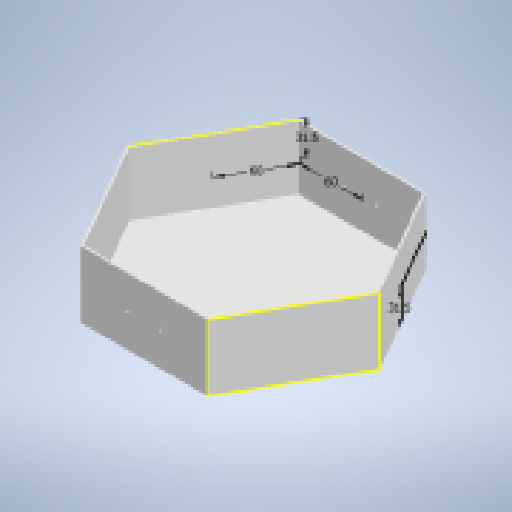
# Autodesk Inventor part: BaseHEX
Saved by Autodesk Inventor 2024 (Build 280153000, 153)
## iProperties
Created: 2024-03-21
Part Number: BaseHEX
Material: Genérico
Document SubType Name: Modeling
Designer: na_re
Density: 1 g/cm^3
Appearance: Valor por defecto
Author: na_re
Autodesk Inventor part; units mm, degrees
ref_plane "YZ Plane" through (0, 0, 0) normal (1, 0, 0) x (0, 1, 0)
ref_plane "XZ Plane" through (0, 0, 0) normal (0, 1, 0) x (-1, 0, 0)
ref_plane "XY Plane" through (0, 0, 0) normal (0, 0, 1) x (1, 0, 0)
sketch "Boceto1" plane through (0, 0, 0) normal (0, 1, 0) x (-1, 0, 0)
  line L0 (120, 0) -> (60, -103.923)
  line L1 (60, -103.923) -> (-60, -103.923)
  line L2 (-60, -103.923) -> (-120, 0)
  line L3 (-120, 0) -> (-60, 103.923)
  line L4 (-60, 103.923) -> (60, 103.923)
  line L5 (60, 103.923) -> (120, 0)
  point P0 (0, 0)
  point P1 (0, 0)
  dimension "d0" = 120
  constraints: 12 end point, 1 coincident, 13 other
  measures "d0" distance of L0.start L0.end
extrude "Extrusión1" add sketch "Boceto1" along normal blind 3
sketch "Boceto2" plane through (0, 3, 0) normal (0, 1, 0) x (1, 0, 0)
  line L0 (-60, -103.923) -> (60, -103.923) projected
  line L1 (60, -103.923) -> (120, 0) projected
  line L2 (120, 0) -> (60, 103.923) projected
  line L3 (60, 103.923) -> (-60, 103.923) projected
  line L4 (-60, 103.923) -> (-120, 0) projected
  line L5 (-120, 0) -> (-60, -103.923) projected
  line L6 (-58.8453, -101.923) -> (58.8453, -101.923)
  line L7 (58.8453, -101.923) -> (117.6906, 0)
  line L8 (117.6906, 0) -> (58.8453, 101.923)
  line L9 (58.8453, 101.923) -> (-58.8453, 101.923)
  line L10 (-58.8453, 101.923) -> (-117.6906, 0)
  line L11 (-117.6906, 0) -> (-58.8453, -101.923)
  point P0 (0, 0)
  dimension "d3" = 2
  constraints: 12 end point, 5 other
  measures "d3" distance between parallel lines of L5 L11
extrude "Extrusión2" add sketch "Boceto2" along normal blind 60
sketch "Boceto5" plane through (120, 0, 0) normal (0.866, 0, 0.5) x (0.5, 0, -0.866)
  line L0 (-120, 0) -> (0, 0) projected
  line L1 (0, 0) -> (0, 63) projected
  line L2 (-120, 63) -> (0, 63) projected
  line L3 (-120, 0) -> (-120, 63) projected
  point P0 (-60, 0)
sketch "Boceto9" plane through (-60, 0, 103.923) normal (-0.866, 0, 0.5) x (0.5, 0, 0.866)
  circle A0 centre (-117, 58.5) radius 1.5 projected
  circle A1 centre (-3, 58.5) radius 1.5 projected
  point P0 (-60, 0)
extrude "Extrusión7" cut sketch "Boceto9" against normal blind 220
sketch "Boceto10" plane through (-120, 0, 0) normal (-0.866, 0, -0.5) x (-0.5, 0, 0.866)
  line L0 (-120, 0) -> (0, 0) projected
  line L1 (0, 0) -> (0, 63) projected
  line L2 (-120, 63) -> (0, 63) projected
  line L3 (-120, 0) -> (-120, 63) projected
  line L4 (-120, 63) -> (-120, 31.5)
  line L5 (-120, 31.5) -> (-60, 31.5)
  line L6 (-60, 31.5) -> (-60, 0)
  dimension "d19" = 31.5
  dimension "d20" = 60
  constraints: 6 end point, 1 midpoint, 1 perpendicular
  measures "d19" distance of L2.start L4.end
  measures "d20" distance of L4.end L5.end
sketch "Boceto12" plane through (60, 0, -103.923) normal (0, 0, -1) x (-1, 0, 0)
  line L0 (120, 0) -> (120, 63) projected
  line L1 (120, 31.5) -> (60, 31.5)
  line L2 (60, 31.5) -> (60, 0)
  dimension "d23" = 60
  constraints: 4 end point, 1 horizontal, 1 midpoint
  measures "d23" distance of L1.start L1.end
sketch "Boceto13" plane through (60, 0, -103.923) normal (0, 0, -1) x (-1, 0, 0)
  circle A0 centre (44.5, 31.5) radius 1.25 projected
  circle A1 centre (75.5, 31.5) radius 1.25 projected
  point P0 (60, 0)
extrude "Extrusión9" cut sketch "Boceto13" against normal blind 220
sketch "Boceto14" plane through (60, 0, -103.923) normal (0.866, 0, -0.5) x (-0.5, 0, -0.866)
  line L0 (-60, 0) -> (-60, 31.5)
  line L1 (-60, 31.5) -> (0, 31.5)
  dimension "d26" = 31.5
  constraints: 4 end point, 1 perpendicular, 1 vertical
  measures "d26" distance of L0.start L0.end
sketch "Boceto15" plane through (60, 0, -103.923) normal (0.866, 0, -0.5) x (-0.5, 0, -0.866)
  circle A0 centre (-75.5, 31.5) radius 1.25 projected
  circle A1 centre (-44.5, 31.5) radius 1.25 projected
  point P0 (-60, 0)
extrude "Extrusión10" cut sketch "Boceto15" against normal blind 220
sketch "Boceto16" plane through (120, 0, 0) normal (0.866, 0, 0.5) x (0.5, 0, -0.866)
  line L0 (-60, 0) -> (-60, 31.5)
  line L1 (-60, 31.5) -> (0, 31.5)
  line L2 (0, 0) -> (0, 63) projected
  dimension "d29" = 31.5
  constraints: 4 end point, 1 midpoint, 1 vertical
  measures "d29" distance of L0.start L0.end
sketch "Boceto17" plane through (120, 0, 0) normal (0.866, 0, 0.5) x (0.5, 0, -0.866)
  circle A0 centre (-75.5, 31.5) radius 1.25 projected
  circle A1 centre (-44.5, 31.5) radius 1.25 projected
  point P0 (-60, 0)
extrude "Extrusión11" cut sketch "Boceto17" against normal blind 220
